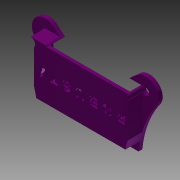
# Autodesk Inventor part: bawahbelakangkecil
Saved by Autodesk Inventor 2015 (Build 190159000, 159)
## iProperties
Created: 2015-01-17
Part Number: bawahbelakangkecil
Material: Generic
Document SubType Name: Modeling
Designer: Rafi Kurnia Putra
Density: 1 g/cm^3
Appearance: Smooth - Purple
Author: Rafi Kurnia Putra
Autodesk Inventor part; units mm, degrees
ref_plane "XY Plane" through (0, 0, 0) normal (0, 0, 1) x (1, 0, 0)
sketch "Sketch1" plane through (0, 0, 0) normal (0, 1, 0) x (-1, 0, 0)
  arc A0 (-40.0744, 9.4382) -> (-43.4, 26.5236) centre (-134.1138, 0) ccw
  line L0 (-43.4, 29.8924) -> (-43.4, 26.5236)
  line L1 (-40.0744, 9.4382) -> (40.0744, 9.4382)
  line L2 (-28.315, 9.4382) -> (28.625, 9.4382)
  line L3 (41.4308, 18.3592) -> (-41.4023, 18.3592)
  arc A1 (55.3297, 52.2069) -> (37.9703, 69.5664) centre (46.665, 60.9016) ccw
  arc A2 (55.3297, 52.2069) -> (40.0744, 9.4382) centre (134.1138, 0) ccw
  line L4 (43.4, 56.6366) -> (43.4, 26.5235)
  line L5 (43.4, 56.6366) -> (43.4, 58.148)
  line L6 (46.65, 65.1366) -> (32.9503, 65.1366)
  line L7 (41.4308, 64.137) -> (31.6221, 64.137)
  line L8 (41.4308, 64.137) -> (43.9118, 64.137)
  arc A3 (31.6221, 64.137) -> (37.9703, 69.5664) centre (0, 107.5366) ccw
  line L9 (-40.0744, 9.4382) -> (40.0744, 9.4382)
  line L10 (40.0744, 18.3592) -> (-40.0744, 18.3592)
  arc A4 (-40.0744, 9.4382) -> (-43.4, 26.5236) centre (-134.1138, 0) ccw
  arc A5 (55.3297, 52.2069) -> (40.0744, 9.4382) centre (135.5613, -0.5163) ccw
  line L11 (-43.4, 26.5236) -> (-43.4, 29.2758)
  arc A6 (-43.4, 26.5236) -> (-55.3297, 52.2069) centre (-134.1138, 0) ccw
  arc A7 (-43.4, 26.5236) -> (-55.3297, 52.2069) centre (-134.1138, 0) ccw
  line L12 (40.5845, 19.3592) -> (-40.5845, 19.3592)
  arc A8 (-40.5845, 19.3592) -> (-42.4402, 26.8042) centre (-134.1138, 0) ccw
  line L13 (42.4, 26.5235) -> (42.4, 56.6366)
  line L14 (42.4, 56.6366) -> (42.4, 58.148)
  line L15 (-42.4, 26.5236) -> (-42.4, 58.148)
  arc A9 (42.4, 26.6664) -> (40.5845, 19.3592) centre (134.1138, 0) ccw
  line L16 (42.4, 58.148) -> (42.4, 60.8866)
  line L17 (0, 41.5801) -> (0, 97.2277) construction
  arc A10 (-37.9703, 69.5664) -> (-31.6221, 64.137) centre (0, 107.5366) ccw
  line L18 (-41.4308, 64.137) -> (-31.6221, 64.137)
  line L19 (-46.65, 65.1366) -> (-32.9503, 65.1366)
  line L20 (-41.4308, 64.137) -> (-43.9118, 64.137)
  arc A11 (-37.9703, 69.5664) -> (-55.3297, 52.2069) centre (-46.665, 60.9016) ccw
  line L21 (-43.4, 56.6366) -> (-43.4, 29.2758)
  arc A12 (-40.0744, 9.4382) -> (-55.3297, 52.2069) centre (-134.1138, 0) ccw
  line L22 (-43.4, 56.6366) -> (-43.4, 26.5235)
  arc A13 (-40.0744, 9.4382) -> (-55.3297, 52.2069) centre (-135.5613, -0.5163) ccw
  line L23 (-42.4, 26.5235) -> (-42.4, 56.6366)
  line L24 (-42.4, 56.6366) -> (-42.4, 58.148)
  arc A14 (-40.5845, 19.3592) -> (-42.4, 26.6664) centre (-134.1138, 0) ccw
  line L25 (-42.4, 58.148) -> (-42.4, 60.8866)
  circle A15 centre (-46.6496, 60.8866) radius 3.25
  arc A16 (-43.3996, 60.8873) -> (-43.4, 29.2758) centre (1113328.4856, 29.363) ccw
  line L26 (-42.4, 60.8866) -> (-42.4, 64.137)
  line L27 (-43.9118, 64.137) -> (-46.65, 64.1366)
  line L28 (-46.65, 65.1366) -> (-46.65, 64.1366)
  line L29 (42.4, 58.148) -> (42.4, 60.8866)
  line L30 (41.4308, 64.137) -> (43.9118, 64.137)
  line L31 (42.4, 56.6366) -> (42.4, 58.148)
  circle A17 centre (46.6496, 60.8866) radius 3.25
  arc A18 (43.4, 29.2758) -> (43.3996, 60.8873) centre (-1113328.4856, 29.344) ccw
  line L32 (42.4, 60.8866) -> (42.4, 64.137)
  line L33 (43.9118, 64.137) -> (46.65, 64.1366)
  line L34 (46.65, 65.1366) -> (46.65, 64.1366)
  circle A19 centre (46.665, 60.9016) radius 3.25
  point P0 (0, 0)
  dimension "d0" = 1
  dimension "d1" = 1
  dimension "d2" = 1
  dimension "d3" = 1
  dimension "d98" = 6.5
  constraints: 70 end point, 47 point on circle, 25 symmetric about line, 20 centre point, 6 point on line, 3 parallel, 2 horizontal, 2 tangent, 1 coincident, 1 collinear, 1 perpendicular, 1 vertical, 8 other
  measures "d0" distance between parallel lines of L3 L12
  measures "d1" radial gap between concentric circles of A0 A8
  measures "d2" distance between parallel lines of L4 L13
  measures "d3" distance between parallel lines of L11 L15
  measures "d98" diameter of A19
extrude "Extrusion1" add sketch "Sketch1" along normal blind 3.5 contours A0 L3 A2 L1 | A17 A19 | A0 L0 L21 A16 A15 L27 L20 L26 L25 L15 A8 L12 A9 L13 L14 L16 L32 L8 L33 A19 A17 A18 L5 L4 A2 L3 | A11 A10 L19 L28 A15 A16 L21 L0 A6 | A10 L18 L20 L27 L28 L19 | L4 L5 A18 A17 A19 L34 L6 A3 A1 A2 | L6 L34 A19 L33 L8 L7 A3 | A19 A17 L34 | L34 L33 A19 | A19 L33 A17 | A17 A19
sketch "Sketch3" plane through (0, 0, 0) normal (0, -1, 0) x (1, 0, 0)
  line L0 (40.5845, 19.3592) -> (41.6059, 19.3592)
  arc A0 (55.3297, 52.2069) -> (40.0744, 9.4382) centre (134.1138, 0) ccw projected
  line L1 (-40.5845, 19.3592) -> (-41.5998, 19.3592)
  line L2 (41.6059, 19.3592) -> (-41.4023, 19.3592)
  line L3 (-41.4023, 18.3592) -> (41.4023, 18.3592)
  arc A1 (41.6059, 19.3592) -> (41.4023, 18.3592) centre (134.1138, 0) ccw
  arc A2 (-40.0744, 9.4382) -> (-55.3297, 52.2069) centre (-134.1138, 0) ccw projected
  arc A3 (-41.4023, 18.3592) -> (-41.6111, 19.3839) centre (-134.1138, 0) ccw
  line L4 (-41.4023, 19.3592) -> (-41.6059, 19.3592)
  line L5 (-41.4023, 19.3592) -> (-41.1986, 19.3592) construction
  point P0 (0, 0)
  dimension "d9" = 180
  constraints: 12 end point, 9 point on circle, 4 horizontal, 2 centre point, 1 collinear, 1 concentric, 1 parallel
  measures "d9" angle of L4 L5
extrude "Extrusion2" add sketch "Sketch3" along normal blind 13.5
sketch "Sketch4" plane through (0, 0, 0) normal (0, -1, 0) x (1, 0, 0)
  line L0 (40.5845, 19.3592) -> (41.6059, 19.3592)
  line L1 (41.6059, 19.3592) -> (-41.6059, 19.3592) projected
  arc A0 (42.4, 26.6664) -> (40.5845, 19.3592) centre (134.1138, 0) ccw
  arc A1 (55.3297, 52.2069) -> (40.0744, 9.4382) centre (134.1138, 0) ccw projected
  arc A2 (43.4419, 26.6664) -> (41.6059, 19.3592) centre (134.1138, 0) ccw
  line L2 (42.4, 58.148) -> (42.4, 60.8866) projected
  line L3 (42.4, 26.6664) -> (42.4, 60.8866)
  line L4 (43.4419, 26.6664) -> (43.4419, 58.099)
  arc A3 (42.4, 60.8866) -> (43.9118, 64.137) centre (46.65, 60.8866) ccw projected
  line L5 (43.4419, 26.6664) -> (74.8746, 26.6664) construction
  arc A4 (42.4, 60.8866) -> (43.4419, 58.099) centre (46.65, 60.8866) ccw
  point P0 (0, 0)
  dimension "d12" = 90
  constraints: 8 end point, 8 point on circle, 3 centre point, 1 collinear, 1 concentric, 1 horizontal, 1 perpendicular
  measures "d12" angle of L5 L4
extrude "Extrusion3" add sketch "Sketch4" along normal blind 13.5
sketch "Sketch5" plane through (0, 0, 0) normal (0, -1, 0) x (1, 0, 0)
  arc A0 (-40.5845, 19.3592) -> (-42.4, 26.6664) centre (-134.1138, 0) ccw
  arc A1 (-41.6059, 19.3592) -> (-55.3297, 52.2069) centre (-134.1138, 0) ccw projected
  arc A2 (-41.6059, 19.3592) -> (-43.4419, 26.6664) centre (-134.1138, 0) ccw
  line L0 (-40.5845, 19.3592) -> (-41.6059, 19.3592)
  line L1 (40.5845, 19.3592) -> (-41.6059, 19.3592) projected
  line L2 (-42.4, 26.6664) -> (-42.4, 60.8866)
  arc A3 (-43.9118, 64.137) -> (-42.4, 60.8866) centre (-46.65, 60.8866) ccw projected
  line L3 (-43.4419, 26.6664) -> (-43.4419, 58.099)
  line L4 (-43.4419, 26.6664) -> (-12.0092, 26.6664) construction
  arc A4 (-43.4419, 58.099) -> (-42.4, 60.8866) centre (-46.65, 60.8866) ccw
  point P0 (0, 0)
  dimension "d15" = 90
  constraints: 8 end point, 8 point on circle, 3 centre point, 1 collinear, 1 concentric, 1 horizontal, 1 perpendicular, 1 tangent, 1 vertical
  measures "d15" angle of L4 L3
extrude "Extrusion4" add sketch "Sketch5" along normal blind 13.5
sketch "Sketch6" plane through (0, 0, 0) normal (0, -1, 0) x (1, 0, 0)
  arc A0 (43.4419, 58.099) -> (43.9118, 64.137) centre (46.65, 60.8866) ccw projected
  line L0 (46.65, 65.1366) -> (32.9503, 65.1366)
  arc A1 (31.6221, 64.137) -> (37.9703, 69.5664) centre (0, 107.5366) ccw projected
  line L1 (43.9118, 64.137) -> (31.6221, 64.137)
  line L2 (42.4, 64.137) -> (31.6221, 64.137) projected
  arc A2 (46.65, 65.1366) -> (43.9118, 64.137) centre (46.65, 60.8866) ccw
  arc A3 (31.6221, 64.137) -> (32.9503, 65.1366) centre (0, 107.5366) ccw
  point P0 (0, 0)
  constraints: 6 point on circle, 4 end point, 2 centre point, 2 concentric, 2 tangent, 1 collinear, 1 horizontal
extrude "Extrusion5" [suppressed]
sketch "Sketch7" plane through (0, 0, 0) normal (0, -1, 0) x (1, 0, 0)
  line L0 (-31.6221, 64.137) -> (-43.9118, 64.137)
  arc A0 (-43.9118, 64.137) -> (-42.4, 60.8866) centre (-46.65, 60.8866) ccw projected
  line L1 (-46.65, 65.1366) -> (-32.9503, 65.1366)
  arc A1 (-37.9703, 69.5664) -> (-31.6221, 64.137) centre (0, 107.5366) ccw projected
  arc A2 (-43.9118, 64.137) -> (-46.65, 65.1366) centre (-46.65, 60.8866) ccw
  arc A3 (-32.9503, 65.1366) -> (-31.6221, 64.137) centre (0, 107.5366) ccw
  point P0 (0, 0)
  constraints: 6 point on circle, 4 end point, 2 centre point, 2 concentric, 2 horizontal, 1 tangent
extrude "Extrusion6" add sketch "Sketch7" along normal blind 13.5
sketch "Sketch8" plane through (0, 0, 0) normal (0, -1, 0) x (1, 0, 0)
  arc A0 (43.9118, 64.137) -> (42.4, 60.8866) centre (46.65, 60.8866) ccw
  arc A1 (43.2676, 64.9018) -> (41.4, 60.8866) centre (46.65, 60.8866) ccw
  line L0 (42.4, 60.8866) -> (42.4, 26.6664) projected
  arc A2 (42.4, 63.9688) -> (42.4, 57.8044) centre (46.65, 60.8866) ccw
  line L1 (42.4, 60.8866) -> (42.4, 57.8044)
  arc A3 (42.4, 60.8866) -> (43.4419, 58.099) centre (46.65, 60.8866) ccw projected
  line L2 (43.9118, 64.137) -> (42.5272, 64.137)
  line L3 (31.6221, 64.137) -> (43.9118, 64.137) projected
  point P0 (0, 0)
  dimension "d22" = 1
  constraints: 8 point on circle, 4 end point, 3 centre point, 2 point on line, 2 tangent, 1 collinear
  measures "d22" radial gap between concentric circles of A0 A1
extrude "Extrusion7" add sketch "Sketch8" along normal blind 13.5
sketch "Sketch9" plane through (0, 0, 0) normal (0, -1, 0) x (1, 0, 0)
  arc A0 (-42.4, 60.8866) -> (-43.9118, 64.137) centre (-46.65, 60.8866) ccw
  arc A1 (-43.9118, 64.137) -> (-42.4, 60.8866) centre (-46.65, 60.8866) ccw projected
  arc A2 (-41.4, 60.8866) -> (-43.2676, 64.9018) centre (-46.65, 60.8866) ccw
  line L0 (-42.4, 26.6664) -> (-42.4, 60.8866) projected
  arc A3 (-42.4, 57.8044) -> (-42.4, 63.9688) centre (-46.65, 60.8866) ccw
  line L1 (-42.4, 60.8866) -> (-42.4, 57.8044)
  line L2 (-31.6221, 64.137) -> (-42.4, 64.137) projected
  line L3 (-42.5272, 64.137) -> (-43.9118, 64.137)
  point P0 (0, 0)
  dimension "d25" = 1
  constraints: 8 point on circle, 4 end point, 3 centre point, 2 collinear, 2 point on line, 1 concentric, 1 tangent
  measures "d25" radial gap between concentric circles of A0 A2
extrude "Extrusion8" add sketch "Sketch9" along normal blind 13.5 contours A0 L3 A2 A3 L0
ref_plane "Work Plane1" through (0, -13.5, 0) normal (0, 1, 0) x (-1, 0, 0)
sketch "Sketch10" plane through (0, -13.5, 0) normal (0, 1, 0) x (-1, 0, 0)
  line L0 (-40.5845, 19.3592) -> (40.5845, 19.3592) projected
  arc A0 (-40.5845, 19.3592) -> (-42.4, 26.6664) centre (-134.1138, 0) ccw projected
  line L1 (-42.4, 57.8044) -> (-42.4, 26.6664) projected
  arc A1 (-42.4, 57.8044) -> (-42.5272, 64.137) centre (-46.65, 60.8866) ccw projected
  line L2 (-31.6221, 64.137) -> (-42.5272, 64.137) projected
  line L3 (42.5272, 64.137) -> (31.6221, 64.137) projected
  arc A2 (42.5272, 64.137) -> (42.4, 57.8044) centre (46.65, 60.8866) ccw projected
  line L4 (42.4, 26.6664) -> (42.4, 57.8044) projected
  arc A3 (42.4, 26.6664) -> (40.5845, 19.3592) centre (134.1138, 0) ccw projected
  line L5 (-31.6221, 64.137) -> (31.6221, 64.137)
  point P0 (0, 0)
  constraints: 2 end point, 1 horizontal
extrude "Extrusion9" add sketch "Sketch10" along normal blind 3.5
sketch "Sketch11" plane through (0, 0, 0) normal (0, 1, 0) x (1, 0, 0)
  arc A0 (42.4, -57.8044) -> (42.4, -63.9688) centre (46.65, -60.8866) ccw projected
  line L0 (42.4, -58.148) -> (42.4, -60.8866) projected
  line L1 (42.4, -57.8044) -> (42.4, -58.148) projected
  arc A1 (42.4, -57.8044) -> (42.4, -63.9688) centre (46.65, -60.8866) ccw projected
  line L2 (42.4, -60.8866) -> (42.4, -63.9688) projected
  point P0 (0, 0)
  point P1 (42.5272, -64.137)
extrude "Extrusion10" add sketch "Sketch11" along normal blind 3.5
sketch "Sketch12" plane through (0, 0, 0) normal (0, 1, 0) x (1, 0, 0)
  line L0 (-42.4, -60.8866) -> (-42.4, -57.8044) projected
  arc A0 (-42.4, -63.9688) -> (-42.4, -57.8044) centre (-46.65, -60.8866) ccw projected
  line L1 (-42.4, -63.9688) -> (-42.4, -60.8866) projected
  point P0 (0, 0)
extrude "Extrusion11" add sketch "Sketch12" along normal blind 3.5
fillet "Fillet1" [suppressed]
fillet "Fillet2" radius 1 1 edges at (0, -10, 64.137)
fillet "Fillet3" [suppressed]
fillet "Fillet4" radius 1 2 edges at (42.4, 1.75, 57.8044) (42.4, -5, 57.8044)
fillet "Fillet5" radius 1 2 edges at (-42.5272, -5, 64.137) (-42.4, -3.25, 57.8044)
fillet "Fillet6" radius 1 9 edges at (-42.4, -3.25, 26.6664) (-40.5845, 1.75, 19.3592) (-40.5845, -5, 19.3592) (0, -10, 19.3592) (-41.4202, -10, 23.0307) (40.5845, -5, 19.3592) (40.5845, 1.75, 19.3592) (42.4, -3.25, 26.6664) (41.4202, -10, 23.0307)
ref_plane "Work Plane2" through (0, 0, 0) normal (1, 0, 0) x (0, 1, 0)
sketch "Sketch15" plane through (0, 0, 0) normal (1, 0, 0) x (0, 1, 0)
  line L0 (0, 52.2069) -> (0, 9.4382) projected
  line L1 (-12.5, 18.3592) -> (0, 18.3592) projected
  line L2 (0, 18.3592) -> (0, 14.2342)
  line L3 (0, 9.4382) -> (0, 9.4382) projected
  line L4 (0, 18.3592) -> (4.125, 18.3592) construction
  line L5 (0, 14.2342) -> (-4.125, 18.3592)
  line L6 (0, 18.3592) -> (-12.5, 18.3592) projected
  line L7 (-4.125, 18.3592) -> (0, 18.3592)
  point P0 (0, 0)
  dimension "d44" = 4.125
  dimension "d45" = 90
  dimension "d46" = 45
  constraints: 8 end point, 1 collinear, 1 horizontal, 1 perpendicular, 1 point on line, 1 vertical, 1 other
  measures "d44" distance of L1.end L2.end
  measures "d45" angle of L2 L4
  measures "d46" angle of L2 L5
extrude "Extrusion12" add sketch "Sketch15" along normal mid plane 50
sketch "Sketch16" plane through (0, -13.5, 0) normal (0, -1, 0) x (1, 0, 0)
  arc A0 (-40.5845, 19.3592) -> (-40.6271, 19.5641) centre (-134.1138, 0) ccw projected
  line L0 (40.7371, 45.6925) -> (40.7371, 37.6925)
  line L1 (40.7371, 37.6925) -> (36.6177, 37.6925)
  spline S0 degree 2 poles (36.6177, 37.6925) (35.4782, 37.6925) (34.2616, 38.0852) (33.5224, 39.1477) (33.5224, 39.91) knots 0 0 0 1 2 3 3 3
  spline S1 degree 2 poles (33.5224, 39.91) (33.5224, 40.5799) (34.0922, 41.5423) (34.585, 41.8426) knots 0 0 0 1 2 2 2
  spline S2 degree 2 poles (34.585, 41.8426) (34.9007, 42.0351) (35.4551, 42.1583) knots 0 0 0 1 1 1
  spline S3 degree 2 poles (35.4551, 42.1583) (35.0162, 42.3046) (34.8083, 42.4509) knots 0 0 0 1 1 1
  spline S4 degree 2 poles (34.8083, 42.4509) (34.6774, 42.551) (34.1615, 43.1978) (34.0691, 43.3749) knots 0 0 0 1 2 2 2
  line L2 (34.0691, 43.3749) -> (32.8756, 45.6925)
  line L3 (32.8756, 45.6925) -> (35.6706, 45.6925)
  line L4 (35.6706, 45.6925) -> (36.9873, 43.244)
  spline S5 degree 2 poles (36.9873, 43.244) (37.2337, 42.7743) (37.4262, 42.628) knots 0 0 0 1 1 1
  spline S6 degree 2 poles (37.4262, 42.628) (37.6957, 42.4432) (38.0345, 42.4432) knots 0 0 0 1 1 1
  line L5 (38.0345, 42.4432) -> (38.25, 42.4432)
  line L6 (38.25, 42.4432) -> (38.25, 45.6925)
  line L7 (38.25, 45.6925) -> (40.7371, 45.6925)
  line L8 (38.25, 40.9341) -> (37.2106, 40.9341)
  spline S7 degree 2 poles (37.2106, 40.9341) (37.0489, 40.9341) (36.5638, 40.8263) knots 0 0 0 1 1 1
  spline S8 degree 2 poles (36.5638, 40.8263) (36.3174, 40.7724) (36.0094, 40.372) (36.0094, 40.1102) knots 0 0 0 1 2 2 2
  spline S9 degree 2 poles (36.0094, 40.1102) (36.0094, 39.7252) (36.4945, 39.3094) (37.1721, 39.3094) knots 0 0 0 1 2 2 2
  line L9 (37.1721, 39.3094) -> (38.25, 39.3094)
  line L10 (38.25, 39.3094) -> (38.25, 40.9341)
  spline S10 degree 2 poles (28.6562, 41.6963) (28.6562, 39.7406) (26.4695, 37.5539) (24.5215, 37.5539) knots 0 0 0 1 2 2 2
  spline S11 degree 2 poles (24.5215, 37.5539) (22.5272, 37.5539) (20.3636, 39.7021) (20.3636, 41.6347) knots 0 0 0 1 2 2 2
  spline S12 degree 2 poles (20.3636, 41.6347) (20.3636, 43.0361) (21.3107, 44.8301) (23.097, 45.8311) (24.4291, 45.8311) knots 0 0 0 1 2 3 3 3
  spline S13 degree 2 poles (24.4291, 45.8311) (25.7765, 45.8311) (27.5551, 44.9687) (28.6562, 43.0977) (28.6562, 41.6963) knots 0 0 0 1 2 3 3 3
  spline S14 degree 2 poles (26.1846, 41.7117) (26.1846, 42.9206) (25.2837, 43.9832) (24.5061, 43.9832) knots 0 0 0 1 2 2 2
  spline S15 degree 2 poles (24.5061, 43.9832) (23.713, 43.9832) (22.8352, 42.9437) (22.8352, 41.6039) knots 0 0 0 1 2 2 2
  spline S16 degree 2 poles (22.8352, 41.6039) (22.8352, 40.4721) (23.7438, 39.4249) (24.5292, 39.4249) knots 0 0 0 1 2 2 2
  spline S17 degree 2 poles (24.5292, 39.4249) (25.276, 39.4249) (26.1846, 40.4875) (26.1846, 41.7117) knots 0 0 0 1 2 2 2
  line L11 (15.2972, 37.6925) -> (10.6697, 37.6925)
  spline S18 degree 2 poles (10.6697, 37.6925) (9.5147, 37.6925) (8.2751, 38.8397) (8.2751, 39.6867) knots 0 0 0 1 2 2 2
  spline S19 degree 2 poles (8.2751, 39.6867) (8.2751, 40.3951) (8.714, 40.9033) knots 0 0 0 1 1 1
  spline S20 degree 2 poles (8.714, 40.9033) (9.0142, 41.2421) (9.584, 41.4422) knots 0 0 0 1 1 1
  spline S21 degree 2 poles (9.584, 41.4422) (8.7217, 41.6501) (7.9055, 42.6588) (7.9055, 43.4211) knots 0 0 0 1 2 2 2
  spline S22 degree 2 poles (7.9055, 43.4211) (7.9055, 44.0371) (8.483, 45.0303) (8.9834, 45.3229) knots 0 0 0 1 2 2 2
  spline S23 degree 2 poles (8.9834, 45.3229) (9.2991, 45.5) (9.9228, 45.5847) knots 0 0 0 1 1 1
  spline S24 degree 2 poles (9.9228, 45.5847) (10.7621, 45.6925) (11.0316, 45.6925) knots 0 0 0 1 1 1
  line L12 (11.0316, 45.6925) -> (15.2972, 45.6925)
  line L13 (15.2972, 45.6925) -> (15.2972, 37.6925)
  line L14 (12.8025, 43.9755) -> (11.5474, 43.9755)
  spline S25 degree 2 poles (11.5474, 43.9755) (10.9084, 43.9755) (10.3848, 43.5212) (10.3848, 43.1439) knots 0 0 0 1 2 2 2
  spline S26 degree 2 poles (10.3848, 43.1439) (10.3848, 42.7897) (10.9007, 42.3585) (11.5474, 42.3585) knots 0 0 0 1 2 2 2
  line L15 (11.5474, 42.3585) -> (12.8025, 42.3585)
  line L16 (12.8025, 42.3585) -> (12.8025, 43.9755)
  line L17 (12.8025, 40.834) -> (11.7322, 40.834)
  spline S27 degree 2 poles (11.7322, 40.834) (11.1548, 40.834) (10.7005, 40.4336) (10.7005, 40.0563) knots 0 0 0 1 2 2 2
  spline S28 degree 2 poles (10.7005, 40.0563) (10.7005, 39.7098) (11.1548, 39.3171) (11.7168, 39.3171) knots 0 0 0 1 2 2 2
  line L18 (11.7168, 39.3171) -> (12.8025, 39.3171)
  line L19 (12.8025, 39.3171) -> (12.8025, 40.834)
  line L20 (-2.3428, 37.6925) -> (-4.8067, 37.6925)
  line L21 (-4.8067, 37.6925) -> (-4.8067, 42.4586)
  spline S29 degree 2 poles (-4.8067, 42.4586) (-4.8067, 43.167) (-4.3679, 44.4297) (-3.4208, 45.3691) (-2.8972, 45.5616) knots 0 0 0 1 2 3 3 3
  spline S30 degree 2 poles (-2.8972, 45.5616) (-2.1811, 45.8311) (-1.1648, 45.8311) knots 0 0 0 1 1 1
  spline S31 degree 2 poles (-1.1648, 45.8311) (-0.5796, 45.8311) (0.7987, 45.6694) (1.7303, 45.1843) (2.5003, 44.2911) (2.6389, 43.8138) knots 0 0 0 1 2 3 4 4 4
  spline S32 degree 2 poles (2.6389, 43.8138) (2.8699, 43.0515) (2.8699, 42.4586) knots 0 0 0 1 1 1
  line L22 (2.8699, 42.4586) -> (2.8699, 37.6925)
  line L23 (2.8699, 37.6925) -> (0.406, 37.6925)
  line L24 (0.406, 37.6925) -> (0.406, 42.5741)
  spline S33 degree 2 poles (0.406, 42.5741) (0.406, 43.2286) (-0.3255, 43.9678) (-0.9723, 43.9678) knots 0 0 0 1 2 2 2
  spline S34 degree 2 poles (-0.9723, 43.9678) (-1.6114, 43.9678) (-2.3428, 43.244) (-2.3428, 42.5741) knots 0 0 0 1 2 2 2
  line L25 (-2.3428, 42.5741) -> (-2.3428, 37.6925)
  line L26 (-9.7346, 43.0438) -> (-12.0907, 42.8975)
  spline S35 degree 2 poles (-12.0907, 42.8975) (-12.1677, 43.475) (-12.3987, 43.7753) knots 0 0 0 1 1 1
  spline S36 degree 2 poles (-12.3987, 43.7753) (-12.7836, 44.2603) (-13.4997, 44.2603) knots 0 0 0 1 1 1
  spline S37 degree 2 poles (-13.4997, 44.2603) (-14.0233, 44.2603) (-14.6008, 43.7599) (-14.6008, 43.4365) knots 0 0 0 1 2 2 2
  spline S38 degree 2 poles (-14.6008, 43.4365) (-14.6008, 43.1285) (-14.3236, 42.8821) knots 0 0 0 1 1 1
  spline S39 degree 2 poles (-14.3236, 42.8821) (-14.0541, 42.6357) (-13.0608, 42.4124) knots 0 0 0 1 1 1
  spline S40 degree 2 poles (-13.0608, 42.4124) (-11.4285, 42.0505) (-10.7355, 41.4422) knots 0 0 0 1 1 1
  spline S41 degree 2 poles (-10.7355, 41.4422) (-10.0348, 40.834) (-10.0348, 39.8946) knots 0 0 0 1 1 1
  spline S42 degree 2 poles (-10.0348, 39.8946) (-10.0348, 39.2786) (-10.7509, 38.1853) (-12.1908, 37.5539) (-13.4381, 37.5539) knots 0 0 0 1 2 3 3 3
  spline S43 degree 2 poles (-13.4381, 37.5539) (-14.9781, 37.5539) (-16.5873, 38.6935) (-16.7413, 39.9408) knots 0 0 0 1 2 2 2
  line L27 (-16.7413, 39.9408) -> (-14.4083, 40.0794)
  spline S44 degree 2 poles (-14.4083, 40.0794) (-14.3159, 39.5404) (-13.7153, 39.0476) (-13.1917, 39.0476) knots 0 0 0 1 2 2 2
  spline S45 degree 2 poles (-13.1917, 39.0476) (-12.7605, 39.0476) (-12.3217, 39.4095) (-12.3217, 39.679) knots 0 0 0 1 2 2 2
  spline S46 degree 2 poles (-12.3217, 39.679) (-12.3217, 39.8638) (-12.5065, 40.0178) knots 0 0 0 1 1 1
  spline S47 degree 2 poles (-12.5065, 40.0178) (-12.6835, 40.1795) (-13.338, 40.3104) knots 0 0 0 1 1 1
  spline S48 degree 2 poles (-13.338, 40.3104) (-14.9627, 40.6646) (-16.364, 41.3807) (-17.0031, 42.4355) (-17.0031, 43.09) knots 0 0 0 1 2 3 3 3
  spline S49 degree 2 poles (-17.0031, 43.09) (-17.0031, 43.86) (-16.1484, 45.1612) (-14.6239, 45.8311) (-13.4535, 45.8311) knots 0 0 0 1 2 3 3 3
  spline S50 degree 2 poles (-13.4535, 45.8311) (-11.4131, 45.8311) (-9.8347, 44.2603) (-9.7346, 43.0438) knots 0 0 0 1 2 2 2
  line L28 (-21.4073, 37.6925) -> (-28.9299, 37.6925)
  line L29 (-28.9299, 37.6925) -> (-28.9299, 39.6713)
  line L30 (-28.9299, 39.6713) -> (-26.4044, 39.6713)
  line L31 (-26.4044, 39.6713) -> (-26.4044, 45.6925)
  line L32 (-26.4044, 45.6925) -> (-23.9328, 45.6925)
  line L33 (-23.9328, 45.6925) -> (-23.9328, 39.6713)
  line L34 (-23.9328, 39.6713) -> (-21.4073, 39.6713)
  line L35 (-21.4073, 39.6713) -> (-21.4073, 37.6925)
  line L36 (-38.6932, 44.3681) -> (-35.8828, 44.3681)
  line L37 (-35.8828, 44.3681) -> (-35.4901, 45.6925)
  line L38 (-35.4901, 45.6925) -> (-32.9646, 45.6925)
  line L39 (-32.9646, 45.6925) -> (-35.9752, 37.6925)
  line L40 (-35.9752, 37.6925) -> (-38.6778, 37.6925)
  line L41 (-38.6778, 37.6925) -> (-41.6807, 45.6925)
  line L42 (-41.6807, 45.6925) -> (-39.0936, 45.6925)
  line L43 (-39.0936, 45.6925) -> (-38.6932, 44.3681)
  line L44 (-38.1773, 42.6357) -> (-37.2995, 39.7637)
  line L45 (-37.2995, 39.7637) -> (-36.4218, 42.6357)
  line L46 (-36.4218, 42.6357) -> (-38.1773, 42.6357)
  point P0 (0, 0)
  point P1 (-0.0406, 41.6925)
  point P2 (-0.0406, 41.6925)
  constraints: 1 centre point, 1 coincident, 1 other
extrude "Extrusion13" cut sketch "Sketch16" against normal through all
sketch "Sketch18" plane through (0, -13.5, 0) normal (0, -1, 0) x (1, 0, 0)
  line L0 (40.7371, 37.6925) -> (40.7371, 45.6925) projected
  line L1 (40.7371, 39.3094) -> (40.7371, 40.9341)
  line L2 (38.25, 40.9341) -> (38.25, 39.3094)
  spline S0 degree 2 poles (24.5061, 43.9832) (23.713, 43.9832) (22.8352, 42.9437) (22.8352, 41.6039) knots 0 0 0 0.5 1 1 1 projected
  spline S1 degree 2 poles (22.8352, 41.6039) (22.8352, 40.4721) (23.7438, 39.4249) (24.5292, 39.4249) knots 0 0 0 0.5 1 1 1 projected
  spline S2 degree 2 poles (24.5292, 39.4249) (25.276, 39.4249) (26.1846, 40.4875) (26.1846, 41.7117) knots 0 0 0 0.5 1 1 1 projected
  spline S3 degree 2 poles (26.1846, 41.7117) (26.1846, 42.9206) (25.2837, 43.9832) (24.5061, 43.9832) knots 0 0 0 0.5 1 1 1 projected
  spline S4 degree 2 poles (28.6562, 41.6963) (28.6562, 39.7406) (26.4695, 37.5539) (24.5215, 37.5539) knots 0 0 0 0.5 1 1 1 projected
  spline S5 degree 2 poles (24.4291, 45.8311) (25.7765, 45.8311) (27.5551, 44.9687) (28.6562, 43.0977) (28.6562, 41.6963) knots 0 0 0 0.333333 0.666667 1 1 1 projected
  spline S6 degree 2 poles (20.3636, 41.6347) (20.3636, 43.0361) (21.3107, 44.8301) (23.097, 45.8311) (24.4291, 45.8311) knots 0 0 0 0.333333 0.666667 1 1 1 projected
  spline S7 degree 2 poles (24.5215, 37.5539) (22.5272, 37.5539) (20.3636, 39.7021) (20.3636, 41.6347) knots 0 0 0 0.5 1 1 1 projected
  line L3 (26.08, 40.6963) -> (28.5753, 40.6963)
  line L4 (26.0856, 42.6963) -> (28.5763, 42.6963)
  line L5 (23.5215, 43.695) -> (23.5215, 45.7654)
  line L6 (25.5215, 43.6589) -> (25.5215, 45.7484)
  line L7 (22.9301, 40.6963) -> (20.4354, 40.6963)
  line L8 (22.9353, 42.6963) -> (20.4428, 42.6963)
  line L9 (28.6562, 41.6963) -> (28.6648, 41.6963) construction
  line L10 (23.5215, 39.7312) -> (23.5215, 37.6305)
  line L11 (24.5215, 45.8306) -> (24.5215, 45.8396)
  line L12 (25.5215, 39.7523) -> (25.5215, 37.6354)
  line L13 (11.7168, 39.3171) -> (12.8025, 39.3171) projected
  line L14 (12.8025, 39.3171) -> (12.8025, 40.834) projected
  line L15 (12.8025, 40.834) -> (11.7322, 40.834) projected
  line L16 (11.5474, 42.3585) -> (12.8025, 42.3585) projected
  line L17 (12.8025, 42.3585) -> (12.8025, 43.9755) projected
  line L18 (12.8025, 43.9755) -> (11.5474, 43.9755) projected
  line L19 (15.2972, 37.6925) -> (15.2972, 45.6925) projected
  line L20 (15.2972, 39.3171) -> (15.2972, 40.834)
  line L21 (12.8025, 40.834) -> (12.8025, 39.3171)
  line L22 (15.2972, 42.3585) -> (15.2972, 43.9755)
  line L23 (12.8025, 43.9755) -> (12.8025, 42.3585)
  line L24 (-35.4901, 45.6925) -> (-35.8828, 44.3681) projected
  line L25 (-35.8828, 44.3681) -> (-36.4218, 42.6357)
  line L26 (-36.4218, 42.6357) -> (-38.1773, 42.6357)
  line L27 (-36.4218, 42.6357) -> (-38.1773, 42.6357) projected
  line L28 (-38.1773, 42.6357) -> (-38.6932, 44.3681)
  line L29 (-38.6932, 44.3681) -> (-35.8828, 44.3681)
  line L30 (-38.6932, 44.3681) -> (-35.8828, 44.3681) projected
  line L31 (12.8025, 39.8255) -> (15.2972, 39.8255)
  line L32 (12.8025, 40.3255) -> (15.2972, 40.3255)
  line L33 (12.8025, 42.917) -> (15.2972, 42.917)
  line L34 (12.8025, 43.417) -> (15.2972, 43.417)
  line L35 (38.25, 39.8717) -> (40.7371, 39.8717)
  line L36 (38.25, 40.3717) -> (40.7371, 40.3717)
  line L37 (38.25, 39.8717) -> (38.25, 40.3717)
  line L38 (38.25, 40.9341) -> (38.25, 39.3094) projected
  line L39 (40.7371, 39.8717) -> (40.7371, 40.3717)
  line L40 (15.2972, 39.8255) -> (15.2972, 40.3255)
  line L41 (12.8025, 39.8255) -> (12.8025, 40.3255)
  line L42 (12.8025, 39.3171) -> (12.8025, 40.834) projected
  line L43 (12.8025, 42.917) -> (12.8025, 43.417)
  line L44 (12.8025, 43.9755) -> (12.8025, 42.3585) projected
  line L45 (15.2972, 42.917) -> (15.2972, 43.417)
  line L46 (40.9871, 39.6217) -> (38, 39.6217)
  line L47 (38, 39.6217) -> (38, 40.6217)
  line L48 (38, 40.6217) -> (40.9871, 40.6217)
  line L49 (40.9871, 40.6217) -> (40.9871, 39.6217)
  line L50 (15.5472, 39.5755) -> (12.5525, 39.5755)
  line L51 (12.5525, 39.5755) -> (12.5525, 40.5755)
  line L52 (12.5525, 40.5755) -> (15.5472, 40.5755)
  line L53 (15.5472, 40.5755) -> (15.5472, 39.5755)
  line L54 (15.5472, 42.667) -> (12.5525, 42.667)
  line L55 (12.5525, 42.667) -> (12.5525, 43.667)
  line L56 (12.5525, 43.667) -> (15.5472, 43.667)
  line L57 (15.5472, 43.667) -> (15.5472, 42.667)
  point P0 (0, 0)
  point P1 (24.5215, 41.6963)
  dimension "d83" = 0.25
  dimension "d84" = 0.25
  dimension "d85" = 0.25
  constraints: 88 end point, 10 parallel, 5 collinear, 3 point on line, 1 horizontal, 1 vertical, 39 other
  measures "d83" distance between parallel lines of L35 L46
  measures "d84" distance between parallel lines of L31 L50
  measures "d85" distance between parallel lines of L33 L54
sketch "Sketch19" plane through (0, -13.5, 0) normal (0, -1, 0) x (1, 0, 0)
  circle A0 centre (24.5076, 41.6963) radius 1
  point P0 (0, 0)
  point P1 (22.9301, 40.6963)
  point P2 (23.5215, 39.7312)
  point P3 (25.5215, 39.7523)
  point P4 (26.08, 40.6963)
  point P5 (26.0856, 42.6963)
  point P6 (25.5215, 43.6589)
  point P7 (23.5215, 43.695)
  point P8 (22.9353, 42.6963)
  constraints: 1 centre point, 4 other
extrude "Extrusion16" cut sketch "Sketch19" against normal through all
extrude "Extrusion18" add sketch "Sketch18" against normal blind 3.5 contours L35 L2 L36 L0 | L0 L48 L49 L46 | L0 L46 L2 L35 | L36 L2 L48 L0 | L2 L46 L47 L48 | S0 L5 S6 S5 L6 S3 | S0 S1 L7 S7 S6 L8 | L4 S5 S4 L3 S2 S3 | S1 S2 L12 S4 S7 L10 | L14 L50 L51 L52 | L31 L19 L50 L14 | L14 L32 L19 L31 | L14 L52 L19 L32 | L19 L52 L53 L50 | L17 L54 L55 L56 | L33 L19 L54 L17 | L17 L34 L19 L33 | L17 L56 L19 L34 | L19 L56 L57 L54 | L25 L26 L28 L29
sketch "Sketch20" plane through (0, -13.5, 0) normal (0, -1, 0) x (1, 0, 0)
  line L0 (-37.2995, 39.7637) -> (-36.4218, 42.6357) projected
  line L1 (-38.1773, 42.6357) -> (-37.2995, 39.7637) projected
  line L2 (-38.6932, 44.3681) -> (-38.1773, 42.6357) projected
  line L3 (-36.4218, 42.6357) -> (-35.8828, 44.3681) projected
  line L4 (-35.8828, 44.3681) -> (-35.4901, 45.6925) projected
  line L5 (-39.0936, 45.6925) -> (-38.6932, 44.3681) projected
  line L6 (-35.4901, 45.6925) -> (-39.0936, 45.6925)
  line L7 (-37.2995, 39.7637) -> (-35.4901, 45.6925)
  line L8 (-37.303, 42.3277) -> (-37.9748, 44.5837)
  line L9 (-37.9748, 44.5837) -> (-38.0833, 44.9425)
  line L10 (-38.0833, 44.9425) -> (-36.4947, 44.9425)
  line L11 (-36.4947, 44.9425) -> (-36.6004, 44.5862)
  line L12 (-36.6004, 44.5862) -> (-37.303, 42.3277)
  point P0 (0, 0)
  dimension "d90" = 0.75
  constraints: 14 end point, 1 horizontal, 4 other
  measures "d90" distance between parallel lines of L2 L8
extrude "Extrusion19" cut sketch "Sketch20" against normal blind 3.5 contours L8 L9 L10 L11 L12
sketch "Sketch23" plane through (0, 3.5, 0) normal (0, 1, 0) x (1, 0, 0)
  circle A0 centre (-46.65, -60.8866) radius 3.25
  point P0 (0, 0)
  dimension "d99" = 6.5
  constraints: 1 centre point, 1 coincident
  measures "d99" diameter of A0
extrude "Extrusion20" cut sketch "Sketch23" against normal through all
body "Solid1"
